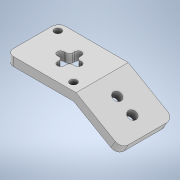
# Autodesk Inventor part: 2번
Saved by Autodesk Inventor 2022 (Build 260153000, 153)
## iProperties
Created: 2021-09-04
Part Number: 2번
Material: 일반
Document SubType Name: Modeling
Designer: 서울공업고등학교
Density: 1 g/cm^3
Appearance: 기본값
Author: 서울공업고등학교
Autodesk Inventor part; units mm, degrees
ref_plane "YZ Plane" through (0, 0, 0) normal (1, 0, 0) x (0, 1, 0)
ref_plane "XZ Plane" through (0, 0, 0) normal (0, 1, 0) x (-1, 0, 0)
ref_plane "XY Plane" through (0, 0, 0) normal (0, 0, 1) x (1, 0, 0)
sketch "스케치1" plane through (0, 0, 0) normal (0, 0, 1) x (1, 0, 0)
  line L0 (0, 0) -> (0, -10)
  line L1 (0, -10) -> (77.3205, -10)
  line L2 (77.3205, -10) -> (126.9615, -38.6603)
  line L3 (126.9615, -38.6603) -> (131.9615, -30)
  line L4 (131.9615, -30) -> (80, 0)
  line L5 (80, 0) -> (0, 0)
  dimension "d0" = 10
  dimension "d1" = 80
  dimension "d2" = 60
  dimension "d4" = 150
  dimension "d5" = 10
  constraints: 12 end point, 2 parallel, 2 perpendicular, 1 vertical
  measures "d0" distance between parallel lines of L1 L5
  measures "d1" distance of L4.end L0.start
  measures "d2" distance of L3.end L4.end
  measures "d4" angle of L2 L1
  measures "d5" distance between parallel lines of L2 L4
extrude "돌출1" add sketch "스케치1" along normal mid plane 60
fillet "모깎기1" radius 8 2 edges at (0, -5, 30) (0, -5, -30)
fillet "모깎기2" radius 8 2 edges at (129.4615, -34.3301, 30) (129.4615, -34.3301, -30)
sketch "스케치2" plane through (80, 0, 30) normal (0.5, 0.866, 0) x (0.866, -0.5, 0)
  circle A0 centre (20, 30) radius 5
  circle A1 centre (40, 30) radius 5
  line L0 (60, 52) -> (60, 8) projected
  line L1 (52, 0) -> (0, 0) projected
  point P0 (-69.282, 30)
  dimension "d10" = 10
  dimension "d11" = 10
  dimension "d12" = 20
  dimension "d13" = 20
  dimension "d14" = 30
  dimension "d15" = 30
  constraints: 2 centre point
  measures "d10" diameter of A0
  measures "d11" diameter of A1
  measures "d12" distance from line of A1.centre L0
  measures "d13" distance of A0.centre A1.centre
  measures "d14" distance from line of A0.centre L1
  measures "d15" distance from line of A1.centre L1
extrude "돌출2" cut sketch "스케치2" against normal blind 60
sketch "스케치3" plane through (80, 0, 30) normal (0, 1, 0) x (1, 0, 0)
  line L0 (-47.6391, 30) -> (-27.6391, 30) construction
  line L1 (-47.6391, 26) -> (-27.6391, 26)
  line L2 (-27.6391, 34) -> (-47.6391, 34)
  arc A0 (-47.6391, 34) -> (-47.6391, 26) centre (-47.6391, 30) ccw
  arc A1 (-27.6391, 26) -> (-27.6391, 34) centre (-27.6391, 30) ccw
  line L3 (-37.6391, 40) -> (-37.6391, 20) construction
  line L4 (-41.6391, 40) -> (-41.6391, 20)
  line L5 (-33.6391, 20) -> (-33.6391, 40)
  arc A2 (-33.6391, 40) -> (-41.6391, 40) centre (-37.6391, 40) ccw
  arc A3 (-41.6391, 20) -> (-33.6391, 20) centre (-37.6391, 20) ccw
  line L6 (-72, 60) -> (0, 60) projected
  circle A4 centre (-72, 51) radius 4
  circle A5 centre (-12, 9) radius 4
  point P0 (-80, 30)
  point P1 (-37.6391, 30)
  point P2 (-37.6391, 30)
  point P3 (-41.6391, 26)
  point P4 (-33.6391, 26)
  point P5 (-33.6391, 34)
  point P6 (-41.6391, 34)
  dimension "d18" = 20
  dimension "d19" = 20
  dimension "d20" = 30
  dimension "d21" = 30
  dimension "d22" = 8
  dimension "d23" = 8
  dimension "d24" = 60
  dimension "d25" = 42
  dimension "d26" = 9
  dimension "d28" = 8
  dimension "d29" = 8
  constraints: 16 end point, 8 point on circle, 8 tangent, 6 centre point, 2 midpoint, 2 parallel, 1 horizontal, 1 vertical
  measures "d18" distance of L3.end L3.start
  measures "d19" distance of L0.end L0.start
  measures "d20" distance from line of L6 point (-37.639, 30)
  measures "d21" distance from line of L6 point (-37.639, 30)
  measures "d22" diameter of A4
  measures "d23" diameter of A5
  measures "d24" horizontal distance of A5.centre A4.centre
  measures "d25" vertical distance of A5.centre A4.centre
  measures "d26" distance from line of L6 A4.centre
  measures "d28" distance between parallel lines of L1 L2
  measures "d29" distance between parallel lines of L5 L4
extrude "돌출3" cut sketch "스케치3" against normal blind 60
fillet "모깎기3" radius 4 4 edges at (38.3609, -5, -4) (38.3609, -5, 4) (46.3609, -5, 4) (46.3609, -5, -4)
